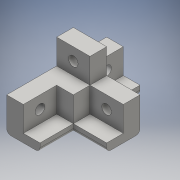
# Autodesk Inventor part: threewayNES
Saved by Autodesk Inventor 2016 (Build 200138000, 138)
## iProperties
Created: 2015-11-25
Part Number: threewayNES
Material: Generic
Document SubType Name: Modeling
Designer: hesaon
Density: 1 g/cm^3
Appearance: Default
Author: hesaon
Autodesk Inventor part; units mm, degrees
ref_plane "YZ Plane" through (0, 0, 0) normal (1, 0, 0) x (0, 1, 0)
ref_plane "XZ Plane" through (0, 0, 0) normal (0, 1, 0) x (-1, 0, 0)
ref_plane "XY Plane" through (0, 0, 0) normal (0, 0, 1) x (1, 0, 0)
sketch "Sketch1" plane through (0, 0, 0) normal (0, 0, 1) x (1, 0, 0)
  line L0 (0, 0) -> (12, 0)
  line L1 (12, 0) -> (12, 12)
  line L2 (12, 12) -> (0, 12)
  line L3 (0, 12) -> (0, 0)
  line L4 (12, 0) -> (0, 0)
  line L5 (0, 0) -> (0, -12)
  line L6 (0, -12) -> (12, -12)
  line L7 (12, -12) -> (12, 0)
  line L8 (12, 0) -> (24, 0)
  line L9 (24, 0) -> (24, -12)
  line L10 (24, -12) -> (12, -12)
  line L11 (12, -12) -> (12, 0)
  line L12 (0, -12) -> (-12, -12)
  line L13 (-12, -12) -> (-12, 0)
  line L14 (-12, 0) -> (0, 0)
  line L15 (0, 0) -> (0, -12)
  line L16 (0, -12) -> (12, -12)
  line L17 (12, -12) -> (12, -24)
  line L18 (12, -24) -> (0, -24)
  line L19 (0, -24) -> (0, -12)
  dimension "d0" = 12
  dimension "d1" = 12
  dimension "d2" = 12
  dimension "d3" = 12
  dimension "d4" = 12
  dimension "d5" = 12
  dimension "d6" = 12
  dimension "d7" = 12
  dimension "d8" = 12
  dimension "d9" = 12
  constraints: 40 end point, 10 parallel, 5 horizontal, 5 perpendicular
  measures "d0" distance of L2.end L1.end
  measures "d1" distance of L1.end L0.end
  measures "d2" distance of L6.end L5.end
  measures "d3" distance of L5.end L4.end
  measures "d4" distance of L9.end L10.end
  measures "d5" distance of L8.end L9.end
  measures "d6" distance of L13.end L14.end
  measures "d7" distance of L12.end L13.end
  measures "d8" distance of L17.end L18.end
  measures "d9" distance of L16.end L17.end
extrude "Extrusion1" add sketch "Sketch1" along normal blind 3
sketch "Sketch2" plane through (0, 0, 3) normal (0, 0, 1) x (1, 0, 0)
  line L0 (-12, 0) -> (-12, -12) projected
  line L1 (-12, -12) -> (-12, -6)
  line L2 (-12, -6) -> (0, -6)
  line L3 (-12, -12) -> (0, -12) projected
  line L4 (0, -6) -> (0, -12)
  line L5 (0, -12) -> (-12, -12)
  line L6 (12, -24) -> (12, -12) projected
  line L7 (12, -12) -> (12, -6)
  line L8 (12, -6) -> (24, -6)
  line L9 (24, -12) -> (24, 0) projected
  line L10 (12, -12) -> (24, -12) projected
  line L11 (24, -6) -> (24, -12)
  line L12 (24, -12) -> (12, -12)
  line L13 (0, 0) -> (0, -6)
  line L14 (12, 0) -> (12, 12) projected
  line L15 (0, 0) -> (12, 0)
  line L16 (12, 0) -> (12, -6)
  line L17 (12, -12) -> (0, -12)
  line L18 (0, 12) -> (0, 0) projected
  line L19 (0, 0) -> (0, 12)
  line L20 (0, 12) -> (6, 12)
  line L21 (12, 12) -> (0, 12) projected
  line L22 (6, 12) -> (6, 0)
  line L23 (6, 0) -> (0, 0)
  line L24 (0, -12) -> (0, -24) projected
  line L25 (0, -12) -> (0, -24)
  line L26 (0, -24) -> (6, -24)
  line L27 (0, -24) -> (12, -24) projected
  line L28 (6, -24) -> (6, -12)
  line L29 (6, -12) -> (0, -12)
  dimension "d12" = 6
  dimension "d13" = 12
  constraints: 40 end point, 6 collinear, 6 midpoint, 5 perpendicular, 2 horizontal, 1 vertical
  measures "d12" distance of L0.end L1.end
  measures "d13" distance of L8.end L7.end
extrude "Extrusion2" add sketch "Sketch2" along normal blind 9 contours L2 L4 L3 L0 | L13 L15 L16 L7 L17 L4 | L17 L28 L26 L24 | L18 L20 L22 L15 | L7 L8 L9 L10
sketch "Sketch3" plane through (0, 0, 12) normal (0, 0, 1) x (1, 0, 0)
  line L0 (0, -6) -> (12, -6)
  line L1 (12, -12) -> (6, -12) projected
  line L2 (12, -6) -> (12, -12)
  line L3 (0, -12) -> (0, -24) projected
  line L4 (12, -12) -> (0, -12)
  line L5 (0, -12) -> (0, -6)
  point P0 (0, 0)
  constraints: 8 end point, 3 perpendicular, 1 horizontal
extrude "Extrusion3" add sketch "Sketch3" along normal blind 9
sketch "Sketch4" plane through (6, -12, 3) normal (0, -1, 0) x (1, 0, 0)
  point P0 (-6, -3)
sketch "Sketch5" plane through (-12, -6, 3) normal (0, 1, 0) x (1, 0, 0)
  circle A0 centre (6, -4.5) radius 1.725
  line L0 (0, 0) -> (0, -9) projected
  line L1 (12, -9) -> (0, -9) projected
  circle A1 centre (18, -13.5) radius 1.725
  line L2 (24, -18) -> (12, -18) projected
  line L3 (24, -9) -> (24, -18) projected
  circle A2 centre (30, -4.5) radius 1.725
  line L4 (36, 0) -> (36, -9) projected
  line L5 (36, -9) -> (24, -9) projected
  point P0 (12, 3)
  dimension "d19" = 3.45
  dimension "d20" = 6
  dimension "d21" = 4.5
  dimension "d22" = 3.45
  dimension "d23" = 4.5
  dimension "d24" = 6
  dimension "d25" = 3.45
  dimension "d26" = 6
  dimension "d27" = 4.5
  constraints: 3 centre point
  measures "d19" diameter of A0
  measures "d20" distance from line of L0 A0.centre
  measures "d21" distance from line of L1 A0.centre
  measures "d22" diameter of A1
  measures "d23" distance from line of L2 A1.centre
  measures "d24" distance from line of L3 A1.centre
  measures "d25" diameter of A2
  measures "d26" distance from line of L4 A2.centre
  measures "d27" distance from line of L5 A2.centre
extrude "Extrusion4" cut sketch "Sketch5" against normal blind 3
sketch "Sketch6" plane through (6, -12, 3) normal (0, -1, 0) x (1, 0, 0)
  circle A0 centre (-12, 4.5) radius 1.725 projected
  line L0 (-10.3546, 7.35) -> (-8.7091, 4.5)
  line L1 (-8.7091, 4.5) -> (-10.3546, 1.65)
  line L2 (-10.3546, 1.65) -> (-13.6454, 1.65)
  line L3 (-13.6454, 1.65) -> (-15.2909, 4.5)
  line L4 (-15.2909, 4.5) -> (-13.6454, 7.35)
  line L5 (-13.6454, 7.35) -> (-10.3546, 7.35)
  circle A1 centre (12, 4.5) radius 1.725 projected
  line L6 (13.6454, 7.35) -> (15.2909, 4.5)
  line L7 (15.2909, 4.5) -> (13.6454, 1.65)
  line L8 (13.6454, 1.65) -> (10.3546, 1.65)
  line L9 (10.3546, 1.65) -> (8.7091, 4.5)
  line L10 (8.7091, 4.5) -> (10.3546, 7.35)
  line L11 (10.3546, 7.35) -> (13.6454, 7.35)
  circle A2 centre (0, 13.5) radius 1.725 projected
  line L12 (1.6454, 16.35) -> (3.2909, 13.5)
  line L13 (3.2909, 13.5) -> (1.6454, 10.65)
  line L14 (1.6454, 10.65) -> (-1.6454, 10.65)
  line L15 (-1.6454, 10.65) -> (-3.2909, 13.5)
  line L16 (-3.2909, 13.5) -> (-1.6454, 16.35)
  line L17 (-1.6454, 16.35) -> (1.6454, 16.35)
  point P0 (-6, -3)
  dimension "d30" = 2.85
  dimension "d31" = 2.85
  dimension "d32" = 2.85
  constraints: 36 end point, 3 coincident, 39 other
  measures "d30" distance from line of L5 point (-12, 4.5)
  measures "d31" distance from line of L11 point (12, 4.5)
  measures "d32" distance from line of L17 point (0, 13.5)
extrude "Extrusion5" cut sketch "Sketch6" against normal blind 3 contours A0 | L0 L1 L2 L3 L4 L5 | A1 | L6 L7 L8 L9 L10 L11 | A2 | L12 L13 L14 L15 L16 L17
sketch "Sketch7" plane through (6, 0, 3) normal (1, 0, 0) x (0, 0, -1)
  circle A0 centre (-4.5, 6) radius 1.725
  circle A1 centre (-4.5, -18) radius 1.725
  line L0 (-9, 0) -> (-9, 12) projected
  line L1 (-9, -24) -> (-9, -12) projected
  line L2 (0, -24) -> (-9, -24) projected
  line L3 (0, 12) -> (-9, 12) projected
  point P0 (3, 0)
  dimension "d35" = 3.45
  dimension "d36" = 3.45
  dimension "d37" = 4.5
  dimension "d38" = 4.5
  dimension "d39" = 6
  dimension "d40" = 6
  constraints: 2 centre point
  measures "d35" diameter of A0
  measures "d36" diameter of A1
  measures "d37" distance from line of L0 A0.centre
  measures "d38" distance from line of L1 A1.centre
  measures "d39" distance from line of L2 A1.centre
  measures "d40" distance from line of L3 A0.centre
extrude "Extrusion6" cut sketch "Sketch7" against normal blind 3
sketch "Sketch8" plane through (0, -6, 3) normal (-1, 0, 0) x (0, 0, 1)
  circle A0 centre (4.5, 12) radius 1.725 projected
  line L0 (1.65, 13.6454) -> (4.5, 15.2909)
  line L1 (4.5, 15.2909) -> (7.35, 13.6454)
  line L2 (7.35, 13.6454) -> (7.35, 10.3546)
  line L3 (7.35, 10.3546) -> (4.5, 8.7091)
  line L4 (4.5, 8.7091) -> (1.65, 10.3546)
  line L5 (1.65, 10.3546) -> (1.65, 13.6454)
  circle A1 centre (4.5, -12) radius 1.725 projected
  line L6 (1.65, -10.3546) -> (4.5, -8.7091)
  line L7 (4.5, -8.7091) -> (7.35, -10.3546)
  line L8 (7.35, -10.3546) -> (7.35, -13.6454)
  line L9 (7.35, -13.6454) -> (4.5, -15.2909)
  line L10 (4.5, -15.2909) -> (1.65, -13.6454)
  line L11 (1.65, -13.6454) -> (1.65, -10.3546)
  point P0 (-3, 6)
  dimension "d43" = 2.85
  dimension "d44" = 2.85
  constraints: 24 end point, 2 coincident, 26 other
  measures "d43" distance from line of L5 point (4.5, 12)
  measures "d44" distance from line of L11 point (4.5, -12)
extrude "Extrusion7" cut sketch "Sketch8" against normal blind 3 contours A0 | L0 L1 L2 L3 L4 L5 | A1 | L6 L7 L8 L9 L10 L11
sketch "Sketch9" plane through (0, 0, 12) normal (0, 0, 1) x (1, 0, 0)
  line L0 (12, 0) -> (12, 12) projected
  line L1 (0, -6) -> (-12, -6) projected
  line L2 (12, 0) -> (0, 0)
  line L3 (0, 0) -> (0, -6)
  line L4 (0, -6) -> (12, -6)
  line L5 (12, -6) -> (12, 0)
  constraints: 8 end point, 2 parallel, 1 horizontal, 1 perpendicular
extrude "Extrusion8" add sketch "Sketch9" along normal blind 9
sketch "Sketch10" plane through (0, 0, 21) normal (0, 0, 1) x (1, 0, 0)
  line L0 (24, -6) -> (12, -6) projected
  line L1 (12, -6) -> (0, -6)
  line L2 (0, -6) -> (0, -12)
  line L3 (0, -12) -> (12, -12)
  line L4 (12, -12) -> (12, -6)
  point P0 (0, 0)
  constraints: 8 end point, 2 parallel, 1 horizontal, 1 perpendicular
sketch "Sketch11" plane through (6, 0, 3) normal (0, 1, 0) x (1, 0, 0)
  circle A0 centre (0, -13.5) radius 1.725 projected
  circle A1 centre (0, -13.5) radius 1.725
  point P0 (-6, 3)
  constraints: 1 centre point, 1 coincident
extrude "Extrusion9" cut sketch "Sketch11" against normal through all
extrude "Extrusion10" cut sketch "Sketch10" against normal blind 9
sketch "Sketch12" plane through (0, 0, 0) normal (0, 0, -1) x (-1, 0, 0)
  line L0 (12, -12) -> (0, -12) projected
  line L1 (12, -12) -> (0, -12)
  line L2 (0, -12) -> (0, 0)
  line L3 (0, 0) -> (12, 0)
  line L4 (12, 0) -> (12, -12)
  constraints: 8 end point, 2 parallel, 1 horizontal, 1 perpendicular
extrude "Extrusion11" cut sketch "Sketch12" against normal through all
sketch "Sketch13" plane through (12, -6, 3) normal (1, 0, 0) x (0, 0, -1)
  line L0 (-9, 0) -> (-18, 0) projected
  line L1 (-9, 0) -> (0, 0)
  line L2 (0, 0) -> (0, 6)
  line L3 (0, 6) -> (-9, 6)
  line L4 (-9, 6) -> (-9, 0)
  point P0 (3, 6)
  constraints: 8 end point, 2 parallel, 1 horizontal, 1 perpendicular
extrude "Extrusion12" add sketch "Sketch13" along normal blind 12
sketch "Sketch15" plane through (24, -12, 0) normal (1, 0, 0) x (0, 0, -1)
  line L0 (-12, 6) -> (-12, 12) projected
  line L1 (0, 0) -> (-12, 0)
  line L2 (-12, 0) -> (-12, 6)
  line L3 (-12, 6) -> (0, 6)
  line L4 (0, 6) -> (0, 0)
  point P0 (0, 12)
  constraints: 8 end point, 2 parallel, 1 horizontal, 1 perpendicular
extrude "Extrusion14" cut sketch "Sketch15" against normal blind 12
sketch "Sketch16" plane through (12, -6, 12) normal (0, -1, 0) x (1, 0, 0)
  circle A0 centre (6, -4.5) radius 1.725 projected
  circle A1 centre (6, -4.5) radius 1.725
  point P0 (-12, -12)
  constraints: 2 coincident, 1 centre point, 1 concentric
extrude "Extrusion15" [suppressed]
sketch "Sketch17" plane through (12, -6, 12) normal (0, -1, 0) x (1, 0, 0)
  line L0 (12, -12) -> (0, -12) projected
  line L1 (0, -12) -> (12, -12)
  line L2 (12, -12) -> (12, -9)
  line L3 (12, -9) -> (0, -9)
  line L4 (0, -9) -> (0, -12)
  point P0 (-12, -12)
  dimension "d64" = 12
  dimension "d65" = 3
  constraints: 8 end point, 2 parallel, 1 horizontal, 1 perpendicular
  measures "d64" distance of L3.end L2.end
  measures "d65" distance of L2.end L1.end
extrude "Extrusion16" add sketch "Sketch17" along normal blind 6
fillet "Fillet2" radius 1.5 5 edges at (18, -12, 0) (12, -18, 0) (18, 0, 0) (12, 6, 0) (0, -6, 0)
sketch "Sketch18" plane through (12, -6, 12) normal (0, -1, 0) x (1, 0, 0)
  circle A0 centre (6, -4.5) radius 1.725 projected
  circle A1 centre (6, -4.5) radius 1.725
  point P0 (-12, -12)
  constraints: 1 centre point, 1 coincident
extrude "Extrusion17" cut sketch "Sketch18" against normal blind 3
sketch "Sketch19" plane through (12, 0, 12) normal (0, 1, 0) x (1, 0, 0)
  point P0 (-12, 12)
sketch "Sketch20" plane through (12, 0, 12) normal (0, 1, 0) x (1, 0, 0)
  circle A0 centre (6, 4.5) radius 1.725 projected
  line L0 (4.3546, 1.65) -> (2.7091, 4.5)
  line L1 (2.7091, 4.5) -> (4.3546, 7.35)
  line L2 (4.3546, 7.35) -> (7.6454, 7.35)
  line L3 (7.6454, 7.35) -> (9.2909, 4.5)
  line L4 (9.2909, 4.5) -> (7.6454, 1.65)
  line L5 (7.6454, 1.65) -> (4.3546, 1.65)
  point P0 (-12, 12)
  dimension "d71" = 5.7
  constraints: 12 end point, 1 coincident, 13 other
  measures "d71" distance between parallel lines of L2 L5
extrude "Extrusion18" cut sketch "Sketch20" against normal blind 3 contours A0 | L0 L1 L2 L3 L4 L5
sketch "Sketch21" plane through (12, 0, 12) normal (0, 1, 0) x (1, 0, 0)
  circle A0 centre (-6, -4.5) radius 1.725 projected
  line L0 (-7.6454, -7.35) -> (-9.2909, -4.5)
  line L1 (-9.2909, -4.5) -> (-7.6454, -1.65)
  line L2 (-7.6454, -1.65) -> (-4.3546, -1.65)
  line L3 (-4.3546, -1.65) -> (-2.7091, -4.5)
  line L4 (-2.7091, -4.5) -> (-4.3546, -7.35)
  line L5 (-4.3546, -7.35) -> (-7.6454, -7.35)
  point P0 (-12, 12)
  dimension "d74" = 5.7
  constraints: 12 end point, 1 coincident, 13 other
  measures "d74" distance between parallel lines of L5 L2
extrude "Extrusion19" cut sketch "Sketch21" against normal blind 3
body "Solid1"
